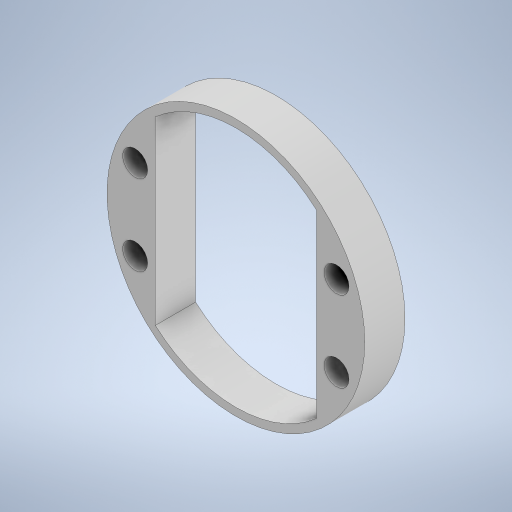
# Autodesk Inventor part: arm_head_back
Saved by Autodesk Inventor 2023.4 (Build 274418000, 418)
## iProperties
Created: 2024-03-10
Part Number: arm_head_back
Material: Generic
Document SubType Name: Modeling
Designer: aaron
Density: 1 g/cm^3
Appearance: Default
Author: aaron
Autodesk Inventor part; units mm, degrees
ref_plane "YZ Plane" through (0, 0, 0) normal (1, 0, 0) x (0, 1, 0)
ref_plane "XZ Plane" through (0, 0, 0) normal (0, 1, 0) x (-1, 0, 0)
ref_plane "XY Plane" through (0, 0, 0) normal (0, 0, 1) x (1, 0, 0)
sketch "Sketch1" plane through (0, 0, 0) normal (0, 0, 1) x (1, 0, 0)
  line L0 (19.067, 0.7556) -> (19.067, 23.1833)
  arc A0 (19.067, 0.7556) -> (19.067, 23.1833) centre (9.067, 11.9694) ccw
  line L1 (-0.933, 23.1833) -> (-0.933, 0.7556)
  arc A1 (-0.933, 23.1833) -> (-0.933, 0.7556) centre (9.067, 11.9694) ccw
  line L2 (12.067, -2.753) -> (12.067, -3.7468)
  arc A2 (12.067, -3.7468) -> (12.067, 27.6857) centre (9.067, 11.9694) ccw
  line L3 (12.067, 27.6857) -> (12.067, 26.6919)
  arc A3 (12.067, -2.753) -> (12.067, 26.6919) centre (9.067, 11.9694) ccw
  line L4 (6.067, -3.7468) -> (6.067, -2.753)
  arc A4 (6.067, 26.6919) -> (6.067, -2.753) centre (9.067, 11.9694) ccw
  line L5 (6.067, 26.6919) -> (6.067, 27.6857)
  arc A5 (6.067, 27.6857) -> (6.067, -3.7468) centre (9.067, 11.9694) ccw
  arc A6 (12.067, 27.6857) -> (6.067, 27.6857) centre (9.067, 11.9694) ccw
  arc A7 (6.067, -3.7468) -> (12.067, -3.7468) centre (9.067, 11.9694) ccw
  circle A8 centre (9.067, 11.9694) radius 15.025
  point P0 (12.067, -2.753)
  point P1 (6.067, -2.753)
  constraints: 16 point on circle, 12 end point, 8 centre point, 1 coincident, 3 other
extrude "Extrusion1" add sketch "Sketch1" along normal blind 5 contours L0 A0 | A0 A3 L3 A2 L2 | L2 A7 L4 A8 | A8 L5 A6 L3 | L4 A5 L5 A4 A1 | A1 L1
sketch "Sketch2" plane through (9.067, 11.9694, 5) normal (0, 0, 1) x (1, 0, 0)
  circle A0 centre (12.5, 5) radius 1.55
  circle A1 centre (12.5, -5) radius 1.55
  circle A2 centre (-12.5, -5) radius 1.55
  circle A3 centre (-12.5, 5) radius 1.55
  circle A4 centre (0, 0) radius 16 projected
  point P0 (-9.067, -11.9694)
  constraints: 4 centre point
extrude "Extrusion2" cut sketch "Sketch2" against normal through all contours A0 | A1 | A2 | A3
body "Solid1"
